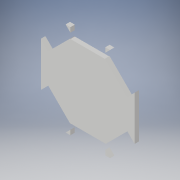
# Autodesk Inventor part: chassis
Saved by Autodesk Inventor 2018 (Build 220112000, 112)
## iProperties
Created: 2018-04-14
Part Number: chassis
Material: Generic
Document SubType Name: Modeling
Designer: dvyen
Density: 1 g/cm^3
Appearance: Default
Author: dvyen
Autodesk Inventor part; units mm, degrees
ref_plane "YZ Plane" through (0, 0, 0) normal (1, 0, 0) x (0, 1, 0)
ref_plane "XZ Plane" through (0, 0, 0) normal (0, 1, 0) x (-1, 0, 0)
ref_plane "XY Plane" through (0, 0, 0) normal (0, 0, 1) x (1, 0, 0)
sketch "Sketch3" plane through (0, 0, 0) normal (0, 0, 1) x (1, 0, 0)
  line L0 (-32, 32) -> (32, 32)
  line L1 (32, 32) -> (32, -32)
  line L2 (32, -32) -> (-32, -32)
  line L3 (-32, -32) -> (-32, 32)
  line L4 (-32, 32) -> (32, -32) construction
  line L5 (32, 32) -> (-32, -32) construction
  line L6 (-32, 32) -> (-15.171, 32)
  line L7 (-15.171, 32) -> (-15.171, 15.171)
  line L8 (-15.171, 15.171) -> (-32, 15.171)
  line L9 (-32, 15.171) -> (-32, 32)
  line L10 (-15.171, 32) -> (-32, 15.171)
  line L11 (32, 32) -> (15.171, 32)
  line L12 (15.171, 32) -> (15.171, 15.171)
  line L13 (15.171, 15.171) -> (32, 15.171)
  line L14 (32, 15.171) -> (32, 32)
  line L15 (15.171, 32) -> (32, 15.171)
  line L16 (-32, -32) -> (-15.171, -32)
  line L17 (-15.171, -32) -> (-15.171, -15.171)
  line L18 (-15.171, -15.171) -> (-32, -15.171)
  line L19 (-32, -15.171) -> (-32, -32)
  line L20 (32, -32) -> (15.171, -32)
  line L21 (15.171, -32) -> (15.171, -15.171)
  line L22 (15.171, -15.171) -> (32, -15.171)
  line L23 (32, -15.171) -> (32, -32)
  line L24 (-32, -15.171) -> (-15.171, -32)
  line L25 (32, -15.171) -> (15.171, -32)
  line L26 (15.171, 32) -> (32, 15.171)
  line L27 (32, 15.171) -> (27.0361, 10.2071)
  line L28 (27.0361, 10.2071) -> (10.2071, 27.0361)
  line L29 (10.2071, 27.0361) -> (15.171, 32)
  line L30 (-15.171, 32) -> (-32, 15.171)
  line L31 (-32, 15.171) -> (-27.0361, 10.2071)
  line L32 (-27.0361, 10.2071) -> (-10.2071, 27.0361)
  line L33 (-10.2071, 27.0361) -> (-15.171, 32)
  line L34 (-32, -15.171) -> (-15.171, -32)
  line L35 (-15.171, -32) -> (-10.2071, -27.0361)
  line L36 (-10.2071, -27.0361) -> (-27.0361, -10.2071)
  line L37 (-27.0361, -10.2071) -> (-32, -15.171)
  line L38 (15.171, -32) -> (32, -15.171)
  line L39 (32, -15.171) -> (27.0361, -10.2071)
  line L40 (27.0361, -10.2071) -> (10.2071, -27.0361)
  line L41 (10.2071, -27.0361) -> (15.171, -32)
  line L42 (-15.171, 22.0722) -> (-22.0722, 15.171)
  line L43 (15.171, 22.0722) -> (22.0722, 15.171)
  line L44 (22.0722, -15.171) -> (15.171, -22.0722)
  line L45 (-15.171, -22.0722) -> (-22.0722, -15.171)
  line L46 (0, 32) -> (11.9, 32)
  line L47 (11.9, 32) -> (-11.9, 32)
  line L48 (-11.9, 32) -> (-11.9, 24.98)
  line L49 (-11.9, 24.98) -> (11.9, 24.98)
  line L50 (11.9, 24.98) -> (11.9, 32)
  line L51 (0, -32) -> (11.9, -32)
  line L52 (11.9, -32) -> (-11.9, -32)
  line L53 (-11.9, -32) -> (-11.9, -24.98)
  line L54 (-11.9, -24.98) -> (11.9, -24.98)
  line L55 (11.9, -24.98) -> (11.9, -32)
  point P0 (0, 0)
  dimension "d21" = 64
  dimension "d22" = 64
  dimension "d23" = 16.829
  dimension "d24" = 16.829
  dimension "d25" = 16.829
  dimension "d26" = 16.829
  dimension "d27" = 16.829
  dimension "d28" = 16.829
  dimension "d29" = 16.829
  dimension "d30" = 16.829
  dimension "d33" = 7.02
  dimension "d34" = 7.02
  dimension "d35" = 7.02
  dimension "d36" = 7.02
  dimension "d37" = 11.9
  dimension "d38" = 23.8
  dimension "d39" = 7.02
  dimension "d40" = 11.9
  dimension "d41" = 23.8
  dimension "d42" = 7.02
  constraints: 112 end point, 25 equal length, 18 point on line, 11 perpendicular, 7 horizontal, 4 midpoint
  measures "d21" distance of L1.end L2.end
  measures "d22" distance of L0.end L1.end
  measures "d23" distance of L7.end L8.end
  measures "d24" distance of L6.end L7.end
  measures "d25" distance of L13.end L12.end
  measures "d26" distance of L12.end L11.end
  measures "d27" distance of L18.end L17.end
  measures "d28" distance of L17.end L16.end
  measures "d29" distance of L21.end L22.end
  measures "d30" distance of L20.end L21.end
  measures "d33" distance of L13.end L27.end
  measures "d34" distance of L31.end L8.end
  measures "d35" distance of L35.end L16.end
  measures "d36" distance of L39.end L22.end
  measures "d37" distance of L46.start L46.end
  measures "d38" distance of L49.end L48.end
  measures "d39" distance of L48.end L47.end
  measures "d40" distance of L51.start L51.end
  measures "d41" distance of L53.end L54.end
  measures "d42" distance of L52.end L53.end
extrude "Extrusion4" add sketch "Sketch3" along normal blind 3 contours L0 L48 L33 | L31 L32 L8 L7 L48 L49 L50 L28 L12 L13 L27 L1 L39 L40 L22 L21 L55 L54 L53 L36 L17 L18 L37 L3 | L7 L8 L32 | L18 L17 L36 | L35 L53 L2 | L0 L29 L50 | L28 L13 L12 | L55 L41 L2 | L40 L21 L22
body "Solid3"
